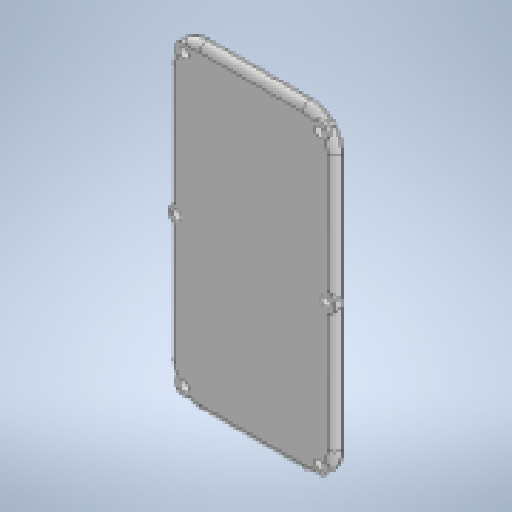
# Autodesk Inventor part: mic-front
Saved by Autodesk Inventor 2025.2 (Build 292293000, 293)
## iProperties
Created: 2025-04-18
Part Number: mic-front
Material: Generic
Document SubType Name: Modeling
Designer: tdeboutte
Density: 1 g/cm^3
Appearance: Default
Author: tdeboutte
Autodesk Inventor part; units mm, degrees
ref_plane "YZ Plane" through (0, 0, 0) normal (1, 0, 0) x (0, 1, 0)
ref_plane "XZ Plane" through (0, 0, 0) normal (0, 1, 0) x (-1, 0, 0)
ref_plane "XY Plane" through (0, 0, 0) normal (0, 0, 1) x (1, 0, 0)
sketch "Sketch1" plane through (0, 0, 0) normal (0, 0, 1) x (1, 0, 0)
  arc A0 (8, 19.3) -> (8, 20.4) centre (8, 19.85) ccw projected
  line L0 (8, 19.3) -> (-8, 19.3) projected
  arc A1 (-8, 20.4) -> (-8, 19.3) centre (-8, 19.85) ccw projected
  line L1 (-8, 20.4) -> (8, 20.4) projected
  arc A2 (-8, 18.7) -> (-8, 17.6) centre (-8, 18.15) ccw projected
  line L2 (-8, 18.7) -> (8, 18.7) projected
  arc A3 (8, 17.6) -> (8, 18.7) centre (8, 18.15) ccw projected
  line L3 (8, 17.6) -> (-8, 17.6) projected
  arc A4 (8, 24.4) -> (8, 25.5) centre (8, 24.95) ccw projected
  line L4 (8, 24.4) -> (-8, 24.4) projected
  arc A5 (-8, 25.5) -> (-8, 24.4) centre (-8, 24.95) ccw projected
  line L5 (-8, 25.5) -> (8, 25.5) projected
  arc A6 (-8, 22.1) -> (-8, 21) centre (-8, 21.55) ccw projected
  line L6 (-8, 22.1) -> (8, 22.1) projected
  arc A7 (8, 21) -> (8, 22.1) centre (8, 21.55) ccw projected
  line L7 (8, 21) -> (-8, 21) projected
  arc A8 (8, 15.9) -> (8, 17) centre (8, 16.45) ccw projected
  line L8 (8, 15.9) -> (-8, 15.9) projected
  arc A9 (-8, 17) -> (-8, 15.9) centre (-8, 16.45) ccw projected
  line L9 (-8, 17) -> (8, 17) projected
  arc A10 (-8, 23.8) -> (-8, 22.7) centre (-8, 23.25) ccw projected
  line L10 (-8, 23.8) -> (8, 23.8) projected
  arc A11 (8, 22.7) -> (8, 23.8) centre (8, 23.25) ccw projected
  line L11 (8, 22.7) -> (-8, 22.7) projected
  arc A12 (-16.5, -2) -> (-16.5, 2) centre (-16.5, 0) ccw projected
  line L12 (-16.5, -28.5) -> (-16.5, -2) projected
  arc A13 (-16.5, -28.5) -> (-16.1383, -30.3671) centre (-11.5, -28.5) ccw projected
  arc A14 (-13.3671, -33.1383) -> (-16.1383, -30.3671) centre (-15.0355, -32.0355) ccw projected
  arc A15 (-13.3671, -33.1383) -> (-11.5, -33.5) centre (-11.5, -28.5) ccw projected
  line L13 (11.5, -33.5) -> (-11.5, -33.5) projected
  arc A16 (11.5, -33.5) -> (13.3671, -33.1383) centre (11.5, -28.5) ccw projected
  arc A17 (16.1383, -30.3671) -> (13.3671, -33.1383) centre (15.0355, -32.0355) ccw projected
  arc A18 (16.1383, -30.3671) -> (16.5, -28.5) centre (11.5, -28.5) ccw projected
  line L14 (16.5, -2) -> (16.5, -28.5) projected
  arc A19 (16.5, 2) -> (16.5, -2) centre (16.5, 0) ccw projected
  line L15 (16.5, 28.5) -> (16.5, 2) projected
  arc A20 (16.5, 28.5) -> (16.1383, 30.3671) centre (11.5, 28.5) ccw projected
  arc A21 (13.3671, 33.1383) -> (16.1383, 30.3671) centre (15.0355, 32.0355) ccw projected
  arc A22 (13.3671, 33.1383) -> (11.5, 33.5) centre (11.5, 28.5) ccw projected
  line L16 (-11.5, 33.5) -> (11.5, 33.5) projected
  arc A23 (-11.5, 33.5) -> (-13.3671, 33.1383) centre (-11.5, 28.5) ccw projected
  arc A24 (-16.1383, 30.3671) -> (-13.3671, 33.1383) centre (-15.0355, 32.0355) ccw projected
  arc A25 (-16.1383, 30.3671) -> (-16.5, 28.5) centre (-11.5, 28.5) ccw projected
  line L17 (-16.5, 2) -> (-16.5, 28.5) projected
  line L18 (-18.5, 28.5) -> (-18.5, -28.5) projected
  arc A26 (-18.5, -28.5) -> (-11.5, -35.5) centre (-11.5, -28.5) ccw projected
  line L19 (-11.5, -35.5) -> (11.5, -35.5) projected
  arc A27 (11.5, -35.5) -> (18.5, -28.5) centre (11.5, -28.5) ccw projected
  line L20 (18.5, -28.5) -> (18.5, 28.5) projected
  arc A28 (18.5, 28.5) -> (11.5, 35.5) centre (11.5, 28.5) ccw projected
  line L21 (11.5, 35.5) -> (-11.5, 35.5) projected
  arc A29 (-11.5, 35.5) -> (-18.5, 28.5) centre (-11.5, 28.5) ccw projected
  line L22 (-16.5, 2) -> (-16.5, 28.5) projected
  arc A30 (-16.1383, 30.3671) -> (-16.5, 28.5) centre (-11.5, 28.5) ccw projected
  arc A31 (-16.1383, 30.3671) -> (-13.3671, 33.1383) centre (-15.0355, 32.0355) ccw projected
  arc A32 (-11.5, 33.5) -> (-13.3671, 33.1383) centre (-11.5, 28.5) ccw projected
  line L23 (-11.5, 33.5) -> (11.5, 33.5) projected
  arc A33 (13.3671, 33.1383) -> (11.5, 33.5) centre (11.5, 28.5) ccw projected
  arc A34 (13.3671, 33.1383) -> (16.1383, 30.3671) centre (15.0355, 32.0355) ccw projected
  arc A35 (16.5, 28.5) -> (16.1383, 30.3671) centre (11.5, 28.5) ccw projected
  line L24 (16.5, 28.5) -> (16.5, 2) projected
  arc A36 (16.5, 2) -> (16.5, -2) centre (16.5, 0) ccw projected
  line L25 (16.5, -2) -> (16.5, -28.5) projected
  arc A37 (16.1383, -30.3671) -> (16.5, -28.5) centre (11.5, -28.5) ccw projected
  arc A38 (16.1383, -30.3671) -> (13.3671, -33.1383) centre (15.0355, -32.0355) ccw projected
  arc A39 (11.5, -33.5) -> (13.3671, -33.1383) centre (11.5, -28.5) ccw projected
  line L26 (11.5, -33.5) -> (-11.5, -33.5) projected
  arc A40 (-13.3671, -33.1383) -> (-11.5, -33.5) centre (-11.5, -28.5) ccw projected
  arc A41 (-13.3671, -33.1383) -> (-16.1383, -30.3671) centre (-15.0355, -32.0355) ccw projected
  arc A42 (-16.5, -28.5) -> (-16.1383, -30.3671) centre (-11.5, -28.5) ccw projected
  line L27 (-16.5, -28.5) -> (-16.5, -2) projected
  arc A43 (-16.5, -2) -> (-16.5, 2) centre (-16.5, 0) ccw projected
  point P0 (0, 0)
extrude "Extrusion1" add sketch "Sketch1" along normal blind 2 contours L0 A1 L1 A0 | L2 A3 L3 A2 | L4 A5 L5 A4 | L6 A7 L7 A6 | L8 A9 L9 A8 | L10 A11 L11 A10 | A12 L17 A25 A24 A23 L16 A22 A21 A20 L15 A19 L14 A18 A17 A16 L13 A15 A14 A13 L12 | A29 L21 A28 L20 A27 L19 A26 L18
fillet "Fillet1" radius 1.6 8 edges at (0, 35.5, 2) (-16.4497, 33.4497, 2) (-18.5, 0, 2) (-16.4497, -33.4497, 2) (0, -35.5, 2) (16.4497, -33.4497, 2) (18.5, 0, 2) (16.4497, 33.4497, 2)
sketch "Sketch2" plane through (0, 0, 0) normal (0, 0, -1) x (-1, 0, 0)
  arc A0 (-16.1383, 30.3671) -> (-13.3671, 33.1383) centre (-15.0355, 32.0355) ccw projected
  arc A1 (13.3671, 33.1383) -> (16.1383, 30.3671) centre (15.0355, 32.0355) ccw projected
  arc A2 (-13.3671, -33.1383) -> (-16.1383, -30.3671) centre (-15.0355, -32.0355) ccw projected
  arc A3 (16.5, 2) -> (16.5, -2) centre (16.5, 0) ccw projected
  arc A4 (-16.5, -2) -> (-16.5, 2) centre (-16.5, 0) ccw projected
  arc A5 (16.1383, -30.3671) -> (13.3671, -33.1383) centre (15.0355, -32.0355) ccw projected
  circle A6 centre (-15.0355, 32.0355) radius 1
  circle A7 centre (15.0355, 32.0355) radius 1
  circle A8 centre (-16.5, 0) radius 1
  circle A9 centre (16.5, 0) radius 1
  circle A10 centre (15.0355, -32.0355) radius 1
  circle A11 centre (-15.0355, -32.0355) radius 1
  point P0 (0, 0)
  dimension "d3" = 2
  dimension "d4" = 2
  dimension "d5" = 2
  dimension "d6" = 2
  dimension "d7" = 2
  dimension "d8" = 2
  constraints: 6 centre point, 6 coincident
  measures "d3" diameter of A6
  measures "d4" diameter of A7
  measures "d5" diameter of A8
  measures "d6" diameter of A9
  measures "d7" diameter of A10
  measures "d8" diameter of A11
extrude "Extrusion2" cut sketch "Sketch2" against normal through all
sketch "Sketch3" plane through (0, 0, 2) normal (0, 0, 1) x (1, 0, 0)
  arc A0 (-16.9, -0.9165) -> (-16.9, 0.9165) centre (-16.5, 0) ccw
  line L0 (-16.9, -28.5) -> (-16.9, -0.9165)
  arc A1 (-16.9, -28.5) -> (-15.9299, -31.5881) centre (-11.5, -28.5) ccw
  arc A2 (-14.5881, -32.9299) -> (-15.9299, -31.5881) centre (-15.0355, -32.0355) ccw
  arc A3 (-14.5881, -32.9299) -> (-11.5, -33.9) centre (-11.5, -28.5) ccw
  line L1 (11.5, -33.9) -> (-11.5, -33.9)
  arc A4 (11.5, -33.9) -> (14.5881, -32.9299) centre (11.5, -28.5) ccw
  arc A5 (15.9299, -31.5881) -> (14.5881, -32.9299) centre (15.0355, -32.0355) ccw
  arc A6 (15.9299, -31.5881) -> (16.9, -28.5) centre (11.5, -28.5) ccw
  line L2 (16.9, -0.9165) -> (16.9, -28.5)
  arc A7 (16.9, 0.9165) -> (16.9, -0.9165) centre (16.5, 0) ccw
  line L3 (16.9, 28.5) -> (16.9, 0.9165)
  arc A8 (16.9, 28.5) -> (15.9299, 31.5881) centre (11.5, 28.5) ccw
  arc A9 (14.5881, 32.9299) -> (15.9299, 31.5881) centre (15.0355, 32.0355) ccw
  arc A10 (14.5881, 32.9299) -> (11.5, 33.9) centre (11.5, 28.5) ccw
  line L4 (-11.5, 33.9) -> (11.5, 33.9)
  arc A11 (-11.5, 33.9) -> (-14.5881, 32.9299) centre (-11.5, 28.5) ccw
  arc A12 (-15.9299, 31.5881) -> (-14.5881, 32.9299) centre (-15.0355, 32.0355) ccw
  arc A13 (-15.9299, 31.5881) -> (-16.9, 28.5) centre (-11.5, 28.5) ccw
  line L5 (-16.9, 0.9165) -> (-16.9, 28.5)
  circle A14 centre (-15.0355, 32.0355) radius 2.0152
  circle A15 centre (15.0355, 32.0355) radius 2.0152
  circle A16 centre (16.5, 0) radius 2.2
  circle A17 centre (15.0355, -32.0355) radius 2
  circle A18 centre (-15.0355, -32.0355) radius 1
  circle A19 centre (-15.0355, -32.0355) radius 2
  circle A20 centre (-16.5, 0) radius 2
  spline S0 degree 6 poles (14.5881, 32.9299) (14.6521, 32.9619) (14.7191, 32.9885) (14.7886, 33.0094) (14.8599, 33.0243) (14.9323, 33.0329) (15.0751, 33.0372) (15.1456, 33.0335) (15.2159, 33.0237) (15.2856, 33.008) (15.354, 32.9862) (15.4793, 32.9339) (15.5367, 32.9047) (15.592, 32.8709) (15.6447, 32.8328) (15.6943, 32.7907) (15.7717, 32.7137) (15.8015, 32.6809) (15.8294, 32.6465) (15.8554, 32.6108) (15.8794, 32.5738) (15.9123, 32.517) (15.9226, 32.4979) (15.9325, 32.4786) (15.9418, 32.459) (15.9506, 32.4393) (15.9863, 32.3535) (16.0079, 32.2857) (16.0235, 32.2167) (16.0332, 32.147) (16.0371, 32.0772) (16.0331, 31.9345) (16.0246, 31.8616) (16.0098, 31.7899) (15.9889, 31.7199) (15.9621, 31.6525) (15.9299, 31.5881) knots 0 0 0 0 0 0 0 0.177555 0.177555 0.177555 0.177555 0.177555 0.347809 0.347809 0.347809 0.347809 0.347809 0.498759 0.498759 0.498759 0.498759 0.498759 0.601645 0.601645 0.601645 0.601645 0.601645 0.652647 0.652647 0.652647 0.652647 0.652647 0.821387 0.821387 0.821387 0.821387 0.821387 1 1 1 1 1 1 1
  arc A21 (16.9, 28.5) -> (15.9299, 31.5881) centre (11.5, 28.5) ccw
  line L6 (18.5, 28.5) -> (16.9, 28.5)
  arc A22 (18.5, 28.5) -> (11.5, 35.5) centre (11.5, 28.5) ccw
  line L7 (11.5, 33.9) -> (11.5, 35.5)
  arc A23 (14.5881, 32.9299) -> (11.5, 33.9) centre (11.5, 28.5) ccw
  arc A24 (-11.5, 35.5) -> (-18.5, 28.5) centre (-11.5, 28.5) ccw
  spline S1 degree 6 poles (-15.9299, 31.5881) (-15.9559, 31.6401) (-15.9783, 31.6941) (-15.9971, 31.7498) (-16.0119, 31.8068) (-16.0226, 31.8648) (-16.0303, 31.9326) (-16.0312, 31.9418) (-16.032, 31.9509) (-16.0328, 31.9601) (-16.0334, 31.9693) (-16.0342, 31.9829) (-16.0344, 31.9873) (-16.0346, 31.9918) (-16.0348, 31.9962) (-16.0349, 32.0007) (-16.0352, 32.0103) (-16.0369, 32.0802) (-16.0328, 32.1506) (-16.0226, 32.2209) (-16.0064, 32.2896) (-15.9842, 32.3588) (-15.9339, 32.4793) (-15.9047, 32.5367) (-15.8709, 32.592) (-15.8328, 32.6447) (-15.7907, 32.6943) (-15.7137, 32.7717) (-15.6809, 32.8015) (-15.6465, 32.8294) (-15.6108, 32.8554) (-15.5738, 32.8794) (-15.517, 32.9123) (-15.4979, 32.9226) (-15.4786, 32.9325) (-15.459, 32.9418) (-15.4393, 32.9506) (-15.3535, 32.9863) (-15.2857, 33.0079) (-15.2167, 33.0235) (-15.147, 33.0332) (-15.0772, 33.0371) (-14.9345, 33.0331) (-14.8616, 33.0246) (-14.7899, 33.0098) (-14.7199, 32.9889) (-14.6525, 32.9621) (-14.5881, 32.9299) knots 0 0 0 0 0 0 0 0.147125 0.147125 0.147125 0.147125 0.147125 0.170022 0.170022 0.170022 0.170022 0.170022 0.180961 0.180961 0.180961 0.180961 0.180961 0.193198 0.350507 0.350507 0.350507 0.350507 0.350507 0.500833 0.500833 0.500833 0.500833 0.500833 0.603293 0.603293 0.603293 0.603293 0.603293 0.654084 0.654084 0.654084 0.654084 0.654084 0.822126 0.822126 0.822126 0.822126 0.822126 1 1 1 1 1 1 1
  arc A25 (-11.5, 33.9) -> (-14.5881, 32.9299) centre (-11.5, 28.5) ccw
  line L8 (-11.5, 35.5) -> (-11.5, 33.9)
  arc A26 (-11.5, 35.5) -> (-18.5, 28.5) centre (-11.5, 28.5) ccw
  line L9 (-18.5, 28.5) -> (-16.9, 28.5)
  arc A27 (-15.9299, 31.5881) -> (-16.9, 28.5) centre (-11.5, 28.5) ccw
  spline S2 degree 6 poles (-16.9, -0.9165) (-16.9373, -0.9002) (-16.9737, -0.8822) (-17.0089, -0.8625) (-17.043, -0.8412) (-17.0758, -0.8186) (-17.1251, -0.7809) (-17.1426, -0.7667) (-17.1596, -0.7522) (-17.1762, -0.7373) (-17.1923, -0.7219) (-17.248, -0.6661) (-17.285, -0.6235) (-17.3188, -0.5789) (-17.3493, -0.5325) (-17.3765, -0.4845) (-17.4661, -0.2991) (-17.5066, -0.1523) (-17.5202, -0.0005) (-17.5068, 0.1521) (-17.4662, 0.2986) (-17.3768, 0.4839) (-17.3497, 0.532) (-17.3192, 0.5784) (-17.2854, 0.623) (-17.2485, 0.6656) (-17.1926, 0.7217) (-17.1763, 0.7371) (-17.1596, 0.7522) (-17.1424, 0.7669) (-17.1247, 0.7812) (-17.0752, 0.8189) (-17.0426, 0.8415) (-17.0086, 0.8627) (-16.9734, 0.8823) (-16.9372, 0.9003) (-16.9, 0.9165) knots 0 0 0 0 0 0 0 0.099017 0.099017 0.099017 0.099017 0.099017 0.155539 0.155539 0.155539 0.155539 0.155539 0.300439 0.300439 0.300439 0.300439 0.300439 0.699286 0.699286 0.699286 0.699286 0.699286 0.844183 0.844183 0.844183 0.844183 0.844183 0.901313 0.901313 0.901313 0.901313 0.901313 1 1 1 1 1 1 1
  line L10 (-16.9, 0.9165) -> (-16.9, 28.5)
  line L11 (-18.5, 28.5) -> (-16.9, 28.5)
  line L12 (-18.5, 28.5) -> (-18.5, -28.5)
  line L13 (-18.5, -28.5) -> (-16.9, -28.5)
  line L14 (-16.9, -28.5) -> (-16.9, -0.9165)
  spline S3 degree 6 poles (16.9, 0.9165) (16.9373, 0.9002) (16.9737, 0.8822) (17.0089, 0.8625) (17.043, 0.8412) (17.0758, 0.8186) (17.1251, 0.7809) (17.1426, 0.7667) (17.1596, 0.7522) (17.1762, 0.7373) (17.1923, 0.7219) (17.248, 0.6661) (17.285, 0.6235) (17.3188, 0.5789) (17.3493, 0.5325) (17.3765, 0.4845) (17.4333, 0.367) (17.4598, 0.2963) (17.4799, 0.2236) (17.4933, 0.1495) (17.5, 0.0748) (17.5, -0.0395) (17.4981, -0.079) (17.4944, -0.1183) (17.4888, -0.1575) (17.4813, -0.1964) (17.4637, -0.2691) (17.454, -0.3031) (17.4428, -0.3367) (17.4302, -0.3698) (17.4161, -0.4024) (17.3674, -0.5034) (17.3277, -0.5696) (17.2815, -0.6326) (17.2291, -0.6917) (17.1707, -0.7461) (17.0752, -0.8189) (17.0426, -0.8415) (17.0086, -0.8627) (16.9734, -0.8823) (16.9372, -0.9003) (16.9, -0.9165) knots 0 0 0 0 0 0 0 0.099066 0.099066 0.099066 0.099066 0.099066 0.155616 0.155616 0.155616 0.155616 0.155616 0.300588 0.300588 0.300588 0.300588 0.300588 0.500248 0.500248 0.500248 0.500248 0.500248 0.605627 0.605627 0.605627 0.605627 0.605627 0.699546 0.699546 0.699546 0.699546 0.699546 0.901435 0.901435 0.901435 0.901435 0.901435 1 1 1 1 1 1 1
  line L15 (16.9, -0.9165) -> (16.9, -28.5)
  line L16 (18.5, -28.5) -> (16.9, -28.5)
  line L17 (18.5, -28.5) -> (18.5, 28.5)
  line L18 (18.5, 28.5) -> (16.9, 28.5)
  line L19 (16.9, 28.5) -> (16.9, 0.9165)
  spline S4 degree 6 poles (15.9299, -31.5881) (15.9619, -31.6521) (15.9885, -31.7191) (16.0094, -31.7886) (16.0243, -31.8599) (16.0329, -31.9323) (16.0372, -32.0751) (16.0335, -32.1456) (16.0237, -32.2159) (16.008, -32.2856) (15.9862, -32.354) (15.9339, -32.4793) (15.9047, -32.5367) (15.8709, -32.592) (15.8328, -32.6447) (15.7907, -32.6943) (15.7137, -32.7717) (15.6809, -32.8015) (15.6465, -32.8294) (15.6108, -32.8554) (15.5738, -32.8794) (15.517, -32.9123) (15.4979, -32.9226) (15.4786, -32.9325) (15.459, -32.9418) (15.4393, -32.9506) (15.3535, -32.9863) (15.2857, -33.0079) (15.2167, -33.0235) (15.147, -33.0332) (15.0772, -33.0371) (14.9345, -33.0331) (14.8616, -33.0246) (14.7899, -33.0098) (14.7199, -32.9889) (14.6525, -32.9621) (14.5881, -32.9299) knots 0 0 0 0 0 0 0 0.177555 0.177555 0.177555 0.177555 0.177555 0.347809 0.347809 0.347809 0.347809 0.347809 0.498759 0.498759 0.498759 0.498759 0.498759 0.601645 0.601645 0.601645 0.601645 0.601645 0.652647 0.652647 0.652647 0.652647 0.652647 0.821387 0.821387 0.821387 0.821387 0.821387 1 1 1 1 1 1 1
  arc A28 (11.5, -33.9) -> (14.5881, -32.9299) centre (11.5, -28.5) ccw
  line L20 (11.5, -35.5) -> (11.5, -33.9)
  arc A29 (11.5, -35.5) -> (18.5, -28.5) centre (11.5, -28.5) ccw
  line L21 (18.5, -28.5) -> (16.9, -28.5)
  arc A30 (15.9299, -31.5881) -> (16.9, -28.5) centre (11.5, -28.5) ccw
  arc A31 (-16.9, -28.5) -> (-15.9299, -31.5881) centre (-11.5, -28.5) ccw
  line L22 (-18.5, -28.5) -> (-16.9, -28.5)
  arc A32 (-18.5, -28.5) -> (-11.5, -35.5) centre (-11.5, -28.5) ccw
  line L23 (-11.5, -35.5) -> (-11.5, -33.9)
  arc A33 (-14.5881, -32.9299) -> (-11.5, -33.9) centre (-11.5, -28.5) ccw
  point P0 (0, 0)
  point P1 (15.9299, -31.5881)
  point P2 (13.6327, -33.461)
  point P3 (16.461, -30.6327)
  point P4 (-16.461, -30.6327)
  point P5 (-13.6327, -33.461)
  point P6 (-13.6176, 33.4675)
  point P7 (-16.2391, 33.6518)
  point P8 (-16.6518, 33.2391)
  point P9 (-16.4675, 30.6176)
  point P10 (15.9299, 31.5881)
  point P11 (16.4675, 30.6176)
  point P12 (16.6518, 33.2391)
  point P13 (16.2391, 33.6518)
  point P14 (13.6176, 33.4675)
  point P15 (16.9, 0.9165)
  point P16 (16.9, -2.1633)
  point P17 (18.5, -0.9165)
  point P18 (18.5, 0.9165)
  point P19 (16.9, 2.1633)
  point P20 (-16.9, -0.9165)
  point P21 (-16.9, 1.9596)
  point P22 (-16.9, -1.9596)
extrude "Extrusion3" add sketch "Sketch3" against normal blind 2 contours L0 A20 L5 S2 | A1 A18 A3 A19 | A14 A24 A11 S1 A13 | A4 S4 A6 A17 | A15 A22 A8 S0 A10 | L2 S3 L3 A16 L17
body "Solid1"
